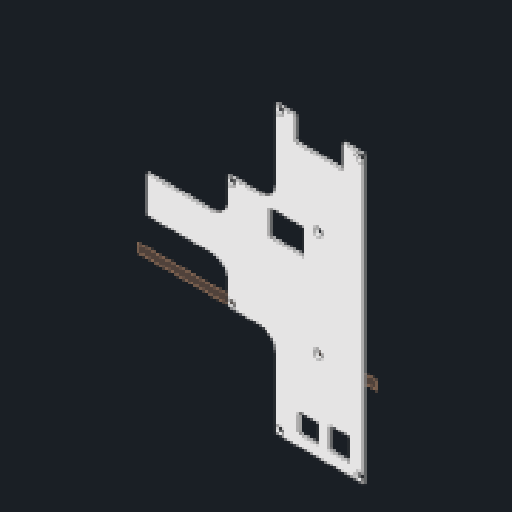
# Autodesk Inventor part: ceil
Saved by Autodesk Inventor 2023 (Build 270158000, 158)
## iProperties
Created: 2024-05-26
Part Number: ceil
Material: ABS Plastic
Document SubType Name: Modeling
Designer: szymo
Density: 1.06 g/cm^3
Appearance: Smooth - White
Mass: 19.0533 g
Surface Area: 253.51 cm^2
Volume: 17.9748 cm^3
Author: szymo
Autodesk Inventor part; units mm, degrees
ref_plane "YZ Plane" through (0, 0, 0) normal (1, 0, 0) x (0, 1, 0)
ref_plane "XZ Plane" through (0, 0, 0) normal (0, 1, 0) x (-1, 0, 0)
ref_plane "XY Plane" through (0, 0, 0) normal (0, 0, 1) x (1, 0, 0)
ref_plane "Work Plane1" through (-50.5, 0, 0) normal (0, 0, 1) x (1, 0, 0)
sketch "Sketch3" plane through (-50.5, 0, 0) normal (0, 0, 1) x (1, 0, 0)
  circle A0 centre (107.3205, 2.5) radius 1.75 projected
  circle A1 centre (53, 2.5) radius 1.75 projected
  line L0 (0, 0) -> (135.5648, 0) projected
  line L1 (135.5648, 0) -> (135.5648, 5) projected
  line L2 (0, 5) -> (135.5648, 5) projected
  line L3 (0, 0) -> (0, 5) projected
  line L4 (0, 24) -> (50.5, 24) projected
  line L5 (50.5, 24) -> (50.5, 28) projected
  line L6 (0, 28) -> (50.5, 28) projected
  line L7 (0, 24) -> (0, 28) projected
  line L8 (0, 47) -> (50.5, 47) projected
  line L9 (0, 47) -> (0, 43) projected
  line L10 (0, 43) -> (50.5, 43) projected
  line L11 (50.5, 47) -> (50.5, 43) projected
  circle A2 centre (107.3205, 68.5) radius 1.75 projected
  circle A3 centre (53, 68.5) radius 1.75 projected
  line L12 (0, 71) -> (135.5648, 71) projected
  line L13 (0, 71) -> (0, 66) projected
  line L14 (0, 66) -> (135.5648, 66) projected
  line L15 (135.5648, 71) -> (135.5648, 66) projected
  arc A4 (130.5648, 120.5) -> (131.5648, 119.5) centre (131.5648, 120.5) ccw projected
  line L16 (131.5648, 119.5) -> (134.5648, 119.5) projected
  arc A5 (134.5648, 119.5) -> (135.5648, 120.5) centre (134.5648, 120.5) ccw projected
  line L17 (135.5648, 124.5) -> (135.5648, 120.5) projected
  line L18 (135.5648, 124.5) -> (50.5, 124.5) projected
  line L19 (50.5, 124.5) -> (50.5, 123.5) projected
  line L20 (50.5, 123.5) -> (80.5, 123.5) projected
  line L21 (80.5, 123.5) -> (80.5, 120.5) projected
  arc A6 (80.5, 120.5) -> (81.5, 119.5) centre (81.5, 120.5) ccw projected
  line L22 (81.5, 119.5) -> (84.5, 119.5) projected
  arc A7 (84.5, 119.5) -> (85.5, 120.5) centre (84.5, 120.5) ccw projected
  line L23 (85.5, 123.5) -> (85.5, 120.5) projected
  line L24 (85.5, 123.5) -> (130.5648, 123.5) projected
  line L25 (130.5648, 123.5) -> (130.5648, 120.5) projected
  circle A8 centre (133.0648, 122) radius 1.75 projected
  circle A9 centre (83, 122) radius 1.75 projected
  line L26 (120.8148, 112) -> (120.8148, 123) projected
  line L27 (120.8148, 123) -> (94.8148, 123) projected
  line L28 (94.8148, 123) -> (94.8148, 112) projected
  line L29 (94.8148, 112) -> (120.8148, 112) projected
  arc A10 (131.5648, -48.5) -> (130.5648, -49.5) centre (131.5648, -49.5) ccw projected
  line L30 (130.5648, -52.5) -> (130.5648, -49.5) projected
  line L31 (85.5, -52.5) -> (130.5648, -52.5) projected
  line L32 (85.5, -52.5) -> (85.5, -49.5) projected
  arc A11 (85.5, -49.5) -> (84.5, -48.5) centre (84.5, -49.5) ccw projected
  line L33 (81.5, -48.5) -> (84.5, -48.5) projected
  arc A12 (81.5, -48.5) -> (80.5, -49.5) centre (81.5, -49.5) ccw projected
  line L34 (80.5, -52.5) -> (80.5, -49.5) projected
  line L35 (50.5, -52.5) -> (80.5, -52.5) projected
  line L36 (50.5, -53.5) -> (50.5, -52.5) projected
  line L37 (135.5648, -53.5) -> (50.5, -53.5) projected
  line L38 (135.5648, -53.5) -> (135.5648, -49.5) projected
  arc A13 (135.5648, -49.5) -> (134.5648, -48.5) centre (134.5648, -49.5) ccw projected
  line L39 (131.5648, -48.5) -> (134.5648, -48.5) projected
  circle A14 centre (133.0648, -51) radius 1.75 projected
  circle A15 centre (83, -51) radius 1.75 projected
  line L40 (95.5648, -45.8) -> (95.5648, -35.2) projected
  line L41 (106.8648, -35.2) -> (95.5648, -35.2) projected
  line L42 (106.8648, -35.2) -> (106.8648, -45.8) projected
  line L43 (95.5648, -45.8) -> (106.8648, -45.8) projected
  circle A16 centre (90.4898, -49.075) radius 1.675 projected
  circle A17 centre (124.5398, -49.075) radius 1.675 projected
  line L44 (126.3648, -33.5) -> (126.3648, -45.5) projected
  line L45 (126.3648, -45.5) -> (114.7648, -45.5) projected
  line L46 (114.7648, -45.5) -> (114.7648, -33.5) projected
  line L47 (114.7648, -33.5) -> (86.8648, -33.5) projected
  line L48 (86.8648, -33.5) -> (86.8648, -52.5) projected
  line L49 (86.8648, -52.5) -> (128.0648, -52.5) projected
  line L50 (128.0648, -52.5) -> (128.0648, -33.5) projected
  line L51 (128.0648, -33.5) -> (126.3648, -33.5) projected
  line L52 (126.3648, -32.7) -> (114.7648, -32.7) projected
  line L53 (114.7648, -32.7) -> (114.7648, -45.5) projected
  line L54 (114.7648, -45.5) -> (126.3648, -45.5) projected
  line L55 (126.3648, -45.5) -> (126.3648, -32.7) projected
  line L56 (80.5, -53.5) -> (135.5648, -53.5)
  line L57 (135.5648, -53.5) -> (135.5648, 124.5)
  line L58 (135.5648, 124.5) -> (80.5, 124.5)
  line L59 (80.5, 124.5) -> (80.5, -53.5)
  line L60 (0, 24) -> (80.5, 24)
  line L61 (80.5, 24) -> (80.5, 47)
  line L62 (80.5, 47) -> (0, 47)
  line L63 (0, 47) -> (0, 24)
  line L64 (80.5, 24) -> (50.5, 24)
  line L65 (50.5, 24) -> (50.5, 0)
  line L66 (50.5, 0) -> (80.5, 0)
  line L67 (80.5, 0) -> (80.5, 24)
  line L68 (50.5, 47) -> (80.5, 47)
  line L69 (80.5, 47) -> (80.5, 71)
  line L70 (80.5, 71) -> (50.5, 71)
  line L71 (50.5, 71) -> (50.5, 47)
  arc A18 (97.9124, 51.3) -> (98.0124, 51.4) centre (97.9124, 51.4) ccw projected
  line L72 (77.4124, 51.3) -> (97.9124, 51.3) projected
  arc A19 (77.3124, 51.4) -> (77.4124, 51.3) centre (77.4124, 51.4) ccw projected
  line L73 (77.3124, 65.9) -> (77.3124, 51.4) projected
  arc A20 (77.4124, 66) -> (77.3124, 65.9) centre (77.4124, 65.9) ccw projected
  line L74 (97.9124, 66) -> (77.4124, 66) projected
  arc A21 (98.0124, 65.9) -> (97.9124, 66) centre (97.9124, 65.9) ccw projected
  line L75 (98.0124, 51.4) -> (98.0124, 65.9) projected
  line L76 (96.2124, 64.1) -> (96.2124, 53.2) projected
  arc A22 (96.2124, 64.1) -> (95.9124, 64.4) centre (95.9124, 64.1) ccw projected
  line L77 (95.9124, 64.4) -> (95.8124, 64.4) projected
  line L78 (95.8124, 64.4) -> (95.3509, 64.95) projected
  line L79 (95.3509, 64.95) -> (94.9739, 64.95) projected
  line L80 (94.9739, 64.95) -> (94.5124, 64.4) projected
  line L81 (94.5124, 64.4) -> (90.8124, 64.4) projected
  line L82 (90.8124, 64.4) -> (90.8124, 64.75) projected
  line L83 (90.8124, 64.75) -> (89.5124, 64.75) projected
  line L84 (89.5124, 64.4) -> (89.5124, 64.75) projected
  line L85 (89.5124, 64.4) -> (85.8124, 64.4) projected
  line L86 (85.8124, 64.4) -> (85.8124, 64.75) projected
  line L87 (85.8124, 64.75) -> (84.5124, 64.75) projected
  line L88 (84.5124, 64.4) -> (84.5124, 64.75) projected
  line L89 (84.5124, 64.4) -> (80.8124, 64.4) projected
  line L90 (80.8124, 64.4) -> (80.3509, 64.95) projected
  line L91 (80.3509, 64.95) -> (79.9739, 64.95) projected
  line L92 (79.9739, 64.95) -> (79.5124, 64.4) projected
  line L93 (79.5124, 64.4) -> (79.4124, 64.4) projected
  arc A23 (79.4124, 64.4) -> (79.1124, 64.1) centre (79.4124, 64.1) ccw projected
  line L94 (79.1124, 64.1) -> (79.1124, 53.2) projected
  arc A24 (79.1124, 53.2) -> (79.4124, 52.9) centre (79.4124, 53.2) ccw projected
  line L95 (79.4124, 52.9) -> (79.5124, 52.9) projected
  line L96 (79.5124, 52.9) -> (79.9739, 52.35) projected
  line L97 (80.3509, 52.35) -> (79.9739, 52.35) projected
  line L98 (80.3509, 52.35) -> (80.8124, 52.9) projected
  line L99 (80.8124, 52.9) -> (84.5124, 52.9) projected
  line L100 (84.5124, 52.9) -> (84.5124, 52.55) projected
  line L101 (85.8124, 52.55) -> (84.5124, 52.55) projected
  line L102 (85.8124, 52.9) -> (85.8124, 52.55) projected
  line L103 (85.8124, 52.9) -> (89.5124, 52.9) projected
  line L104 (89.5124, 52.9) -> (89.5124, 52.55) projected
  line L105 (90.8124, 52.55) -> (89.5124, 52.55) projected
  line L106 (90.8124, 52.9) -> (90.8124, 52.55) projected
  line L107 (90.8124, 52.9) -> (94.5124, 52.9) projected
  line L108 (94.5124, 52.9) -> (94.9739, 52.35) projected
  line L109 (95.3509, 52.35) -> (94.9739, 52.35) projected
  line L110 (95.3509, 52.35) -> (95.8124, 52.9) projected
  line L111 (95.8124, 52.9) -> (95.9124, 52.9) projected
  arc A25 (95.9124, 52.9) -> (96.2124, 53.2) centre (95.9124, 53.2) ccw projected
  line L112 (78.1624, 55.75) -> (78.8624, 55.75) projected
  line L113 (78.8624, 55.75) -> (78.8624, 61.55) projected
  line L114 (78.1624, 61.55) -> (78.8624, 61.55) projected
  line L115 (78.1624, 61.55) -> (78.1624, 55.75) projected
  line L116 (97.1624, 61.55) -> (97.1624, 55.75) projected
  line L117 (96.4624, 61.55) -> (97.1624, 61.55) projected
  line L118 (96.4624, 55.75) -> (96.4624, 61.55) projected
  line L119 (96.4624, 55.75) -> (97.1624, 55.75) projected
  arc A26 (76.8124, 51.4) -> (77.4124, 50.8) centre (77.4124, 51.4) ccw
  line L120 (77.4124, 50.8) -> (97.9124, 50.8)
  arc A27 (97.9124, 50.8) -> (98.5124, 51.4) centre (97.9124, 51.4) ccw
  line L121 (98.5124, 51.4) -> (98.5124, 65.9)
  arc A28 (98.5124, 65.9) -> (97.9124, 66.5) centre (97.9124, 65.9) ccw
  line L122 (97.9124, 66.5) -> (77.4124, 66.5)
  arc A29 (77.4124, 66.5) -> (76.8124, 65.9) centre (77.4124, 65.9) ccw
  line L123 (76.8124, 65.9) -> (76.8124, 51.4)
  line L124 (95.0648, -34.7) -> (95.0648, -46.3)
  line L125 (95.0648, -46.3) -> (107.3648, -46.3)
  line L126 (107.3648, -46.3) -> (107.3648, -34.7)
  line L127 (107.3648, -34.7) -> (95.0648, -34.7)
  line L128 (114.2648, -45.5) -> (114.2648, -32.2)
  line L129 (114.2648, -32.2) -> (126.8648, -32.2)
  line L130 (126.8648, -32.2) -> (126.8648, -45.5)
  line L131 (126.3648, -46) -> (114.7648, -46)
  line L132 (92.8148, 110) -> (92.8148, 125)
  line L133 (92.8148, 125) -> (122.8148, 125)
  line L134 (122.8148, 125) -> (122.8148, 110)
  line L135 (122.8148, 110) -> (92.8148, 110)
  line L136 (114.2648, -45.5) -> (114.2648, -46)
  line L137 (114.2648, -46) -> (114.7648, -46)
  line L138 (126.3648, -46) -> (126.8648, -46)
  line L139 (126.8648, -46) -> (126.8648, -45.5)
  point P0 (122.8148, 124.5)
  point P1 (92.8148, 124.5)
  point P2 (80.5, 0)
  dimension "d16" = 0.5
  dimension "d17" = 0.5
  dimension "d18" = 0.5
  dimension "d19" = 0.5
  dimension "d20" = 2
  constraints: 72 end point, 9 parallel, 8 point on circle, 6 perpendicular, 5 point on line, 4 centre point, 4 horizontal, 2 collinear, 1 vertical, 15 other
  measures "d16" distance between parallel lines of L73 L123
  measures "d17" distance between parallel lines of L40 L124
  measures "d18" distance between parallel lines of L53 L128
  measures "d19" distance between parallel lines of L45 L131
  measures "d20" distance between parallel lines of L28 L132
extrude "Extrusion2" add sketch "Sketch3" along normal blind 1.5 contours A0 | A1 | L65 L2 L59 L0 | L59 L2 L1 L0 | L0 L57 A13 L39 A10 L30 L31 L50 L51 L130 L129 L128 L47 L48 L32 A11 L33 A12 L59 | L65 L60 L59 L2 | A12 L33 A11 L32 L31 L30 A10 L39 A13 L38 L37 L59 L34 | L59 L120 A27 L121 A28 L14 L57 L2 | L4 L7 L6 L5 | L5 L6 L63 L10 L11 L62 L59 L60 | L14 A28 L122 L59 L12 L15 | L62 L71 L14 A29 L123 A26 L120 L59 | L12 L59 A6 L22 A7 L23 L24 L132 L135 L134 L25 A4 L16 A5 L57 | L11 L10 L9 L8 | L59 L122 A29 L14 L71 L12 | A5 L16 A4 L25 L24 L134 L18 L17 | L21 L59 L18 L132 L24 L23 A7 L22 A6 | L48 L47 L128 L136 L137 L131 L138 L139 L130 L51 L50 L31 | A2 | A3 | A8 | A9 | A14 | A15 | A16 | A17
fillet "Fillet2" radius 1 10 edges at (44.5648, -46.3, 0.75) (44.5648, -34.7, 0.75) (56.8648, -34.7, 0.75) (56.8648, -46.3, 0.75) (63.7648, -46, 0.75) (63.7648, -32.2, 0.75) (76.3648, -32.2, 0.75) (76.3648, -46, 0.75) (42.3148, 110, 0.75) (72.3148, 110, 0.75)
fillet "Fillet3" radius 10 4 edges at (30, 0, 0.75) (0, 24, 0.75) (0, 47, 0.75) (30, 71, 0.75)
sketch "Sketch4" plane through (-50.5, 0, 1.5) normal (0, 0, 1) x (1, 0, 0)
  arc A0 (131.5648, -48.5) -> (130.5648, -49.5) centre (131.5648, -49.5) ccw projected
  line L0 (130.5648, -52.5) -> (130.5648, -49.5) projected
  line L1 (85.5, -52.5) -> (130.5648, -52.5) projected
  line L2 (85.5, -52.5) -> (85.5, -49.5) projected
  arc A1 (85.5, -49.5) -> (84.5, -48.5) centre (84.5, -49.5) ccw projected
  line L3 (81.5, -48.5) -> (84.5, -48.5) projected
  arc A2 (81.5, -48.5) -> (80.5, -49.5) centre (81.5, -49.5) ccw projected
  line L4 (80.5, -52.5) -> (80.5, -49.5) projected
  line L5 (50.5, -52.5) -> (80.5, -52.5) projected
  line L6 (50.5, -53.5) -> (50.5, -52.5) projected
  line L7 (135.5648, -53.5) -> (50.5, -53.5) projected
  line L8 (135.5648, -53.5) -> (135.5648, -49.5) projected
  arc A3 (135.5648, -49.5) -> (134.5648, -48.5) centre (134.5648, -49.5) ccw projected
  line L9 (131.5648, -48.5) -> (134.5648, -48.5) projected
  circle A4 centre (133.0648, -51) radius 1.75 projected
  circle A5 centre (83, -51) radius 1.75 projected
  arc A6 (130.5648, 120.5) -> (131.5648, 119.5) centre (131.5648, 120.5) ccw projected
  line L10 (131.5648, 119.5) -> (134.5648, 119.5) projected
  arc A7 (134.5648, 119.5) -> (135.5648, 120.5) centre (134.5648, 120.5) ccw projected
  line L11 (135.5648, 124.5) -> (135.5648, 120.5) projected
  line L12 (135.5648, 124.5) -> (50.5, 124.5) projected
  line L13 (50.5, 124.5) -> (50.5, 123.5) projected
  line L14 (50.5, 123.5) -> (80.5, 123.5) projected
  line L15 (80.5, 123.5) -> (80.5, 120.5) projected
  arc A8 (80.5, 120.5) -> (81.5, 119.5) centre (81.5, 120.5) ccw projected
  line L16 (81.5, 119.5) -> (84.5, 119.5) projected
  arc A9 (84.5, 119.5) -> (85.5, 120.5) centre (84.5, 120.5) ccw projected
  line L17 (85.5, 123.5) -> (85.5, 120.5) projected
  line L18 (85.5, 123.5) -> (130.5648, 123.5) projected
  line L19 (130.5648, 123.5) -> (130.5648, 120.5) projected
  circle A10 centre (133.0648, 122) radius 1.75 projected
  circle A11 centre (83, 122) radius 1.75 projected
  circle A12 centre (107.3205, 68.5) radius 1.75 projected
  circle A13 centre (53, 68.5) radius 1.75 projected
  line L20 (0, 71) -> (135.5648, 71) projected
  line L21 (0, 71) -> (0, 66) projected
  line L22 (0, 66) -> (135.5648, 66) projected
  line L23 (135.5648, 71) -> (135.5648, 66) projected
  circle A14 centre (107.3205, 2.5) radius 1.75 projected
  circle A15 centre (53, 2.5) radius 1.75 projected
  line L24 (0, 0) -> (135.5648, 0) projected
  line L25 (135.5648, 0) -> (135.5648, 5) projected
  line L26 (0, 5) -> (135.5648, 5) projected
  line L27 (0, 0) -> (0, 5) projected
  line L28 (0, 24) -> (50.5, 24) projected
  line L29 (50.5, 24) -> (50.5, 28) projected
  line L30 (0, 28) -> (50.5, 28) projected
  line L31 (0, 24) -> (0, 28) projected
  line L32 (0, 47) -> (50.5, 47) projected
  line L33 (0, 47) -> (0, 43) projected
  line L34 (0, 43) -> (50.5, 43) projected
  line L35 (50.5, 47) -> (50.5, 43) projected
  point P0 (50.5, 0)
  constraints: 8 coincident
hole "Hole2" at (32.5, -51, 1.5) at (82.5648, -51, 1.5) at (82.5648, 122, 1.5) at (32.5, 122, 1.5) at (56.8205, 68.5, 1.5) at (56.8205, 2.5, 1.5) at (2.5, 2.5, 1.5) at (2.5, 68.5, 1.5) direction (0, 0, -1) diameter 2.9 end through all countersink diameter 5.5 countersink angle 90 clearance for "Countersunk Flat Head Screw ISO 2009/7046" size "M2.5" standard "ISO"
body "Solid2"
